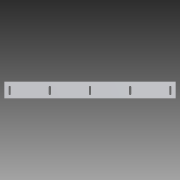
# Autodesk Inventor part: 26in Angle Channel
Saved by Autodesk Inventor 2013 (Build 170138000, 138)
## iProperties
Created: 2013-01-27
Part Number: 26in Angle Channel
Material: Aluminum 6061
Document SubType Name: Modeling
Designer: Naphat
Density: 2.71 g/cm^3
Mass: 398.799 g
Surface Area: 1027.21 cm^2
Volume: 147.158 cm^3
Author: Naphat
Autodesk Inventor part; units mm, degrees
ref_plane "YZ Plane" through (0, 0, 0) normal (1, 0, 0) x (0, 1, 0)
ref_plane "XZ Plane" through (0, 0, 0) normal (0, 1, 0) x (-1, 0, 0)
ref_plane "XY Plane" through (0, 0, 0) normal (0, 0, 1) x (1, 0, 0)
sketch "Sketch1" plane through (0, 0, 0) normal (0, 1, 0) x (-1, 0, 0)
  line L0 (0, 0) -> (50, 0)
  line L1 (50, 0) -> (50, 3)
  line L2 (0, 0) -> (0, 50)
  line L3 (0, 50) -> (3, 50)
  line L4 (3, 50) -> (3, 3)
  line L5 (3, 3) -> (50, 3)
  dimension "d0" = 50
  dimension "d1" = 3
  dimension "d2" = 50
  dimension "d3" = 3
  constraints: 12 end point, 3 perpendicular, 2 parallel, 1 horizontal
  measures "d0" distance of L0.start L0.end
  measures "d1" distance of L0.end L1.end
  measures "d2" distance of L0.start L2.end
  measures "d3" distance of L2.end L3.end
extrude "Extrusion1" add sketch "Sketch1" along normal blind 514.4008
sketch "Sketch2" plane through (-3, 0, 3) normal (-1, 0, 0) x (0, 0, 1)
  line L0 (0, 514.4008) -> (47, 514.4008) projected
  line L1 (0, 0) -> (47, 0) projected
  line L2 (47, 0) -> (47, 514.4008) projected
  line L3 (0, 0) -> (0, 514.4008) projected
  line L4 (-3, 0) -> (-3, 514.4008) projected
  line L5 (-3, 0) -> (0, 0) projected
  line L6 (-3, 514.4008) -> (0, 514.4008) projected
  line L7 (12.7, 498.4008) -> (34.3, 498.4008) construction
  line L8 (12.7, 501.5758) -> (34.3, 501.5758)
  line L9 (12.7, 495.2258) -> (34.3, 495.2258)
  arc A0 (12.7, 501.5758) -> (12.7, 495.2258) centre (12.7, 498.4008) ccw
  arc A1 (34.3, 495.2258) -> (34.3, 501.5758) centre (34.3, 498.4008) ccw
  line L10 (12.7, 19.175) -> (34.3, 19.175)
  line L11 (34.3, 12.825) -> (12.7, 12.825)
  line L12 (12.7, 16) -> (34.3, 16) construction
  arc A2 (12.7, 19.175) -> (12.7, 12.825) centre (12.7, 16) ccw
  arc A3 (34.3, 12.825) -> (34.3, 19.175) centre (34.3, 16) ccw
  line L13 (12.7, 136.6002) -> (34.3, 136.6002) construction
  line L14 (12.7, 139.7752) -> (34.3, 139.7752)
  line L15 (12.7, 133.4252) -> (34.3, 133.4252)
  arc A4 (12.7, 139.7752) -> (12.7, 133.4252) centre (12.7, 136.6002) ccw
  arc A5 (34.3, 133.4252) -> (34.3, 139.7752) centre (34.3, 136.6002) ccw
  line L16 (12.7, 377.8006) -> (34.3, 377.8006) construction
  line L17 (12.7, 380.9756) -> (34.3, 380.9756)
  line L18 (12.7, 374.6256) -> (34.3, 374.6256)
  arc A6 (12.7, 380.9756) -> (12.7, 374.6256) centre (12.7, 377.8006) ccw
  arc A7 (34.3, 374.6256) -> (34.3, 380.9756) centre (34.3, 377.8006) ccw
  line L19 (12.7, 257.2004) -> (34.3, 257.2004) construction
  line L20 (12.7, 260.3754) -> (34.3, 260.3754)
  line L21 (12.7, 254.0254) -> (34.3, 254.0254)
  arc A8 (12.7, 260.3754) -> (12.7, 254.0254) centre (12.7, 257.2004) ccw
  arc A9 (34.3, 254.0254) -> (34.3, 260.3754) centre (34.3, 257.2004) ccw
  dimension "d58" = 12.7
  dimension "d59" = 12.7
  dimension "d60" = 3.175
  dimension "d61" = 6.35
  dimension "d62" = 6.35
  dimension "d63" = 3.175
  dimension "d70" = 16
  dimension "d73" = 16
  dimension "d74" = 3.175
  dimension "d75" = 6.35
  dimension "d76" = 3.175
  dimension "d77" = 6.35
  dimension "d78" = 3.175
  dimension "d79" = 6.35
  dimension "d80" = 482.4008
  dimension "d81" = 120.6002
  dimension "d82" = 120.6002
  dimension "d83" = 120.6002
  constraints: 30 end point, 20 point on circle, 12 parallel, 10 centre point, 10 coincident, 9 tangent, 8 vertical alignment, 1 equal radius
  measures "d58" distance from line of L3 L7.start
  measures "d59" distance from line of L7.end L2
  measures "d60" distance between parallel lines of L8 L7
  measures "d61" distance between parallel lines of L8 L9
  measures "d62" distance of L10.end L11.start
  measures "d63" distance between parallel lines of L10 L12
  measures "d70" distance between parallel lines of L1 L12
  measures "d73" distance between parallel lines of L7 L0
  measures "d74" distance between parallel lines of L14 L13
  measures "d75" distance between parallel lines of L14 L15
  measures "d76" distance between parallel lines of L17 L16
  measures "d77" distance between parallel lines of L17 L18
  measures "d78" distance between parallel lines of L20 L19
  measures "d79" distance between parallel lines of L20 L21
  measures "d80" distance between parallel lines of L7 L12
  measures "d81" distance between parallel lines of L13 L12
  measures "d82" distance between parallel lines of L19 L13
  measures "d83" distance between parallel lines of L16 L19
extrude "Extrusion3" cut sketch "Sketch2" against normal blind 3 contours L8 A1 L9 A0 | L10 A3 L11 A2 | L14 A5 L15 A4 | L17 A7 L18 A6 | L20 A9 L21 A8
equation "\"d73\" = d70"
equation "\"d81\" = 0.25 * d80"
equation "\"d82\" = d81"
equation "\"d83\" = d82"
body "Solid1"
